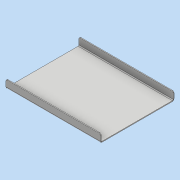
# Autodesk Inventor part: Schale
Saved by Autodesk Inventor 2018 (Build 220112000, 112)
## iProperties
Created: 2020-10-04
Part Number: Schale
Material: Generisch
Document SubType Name: Blech
Designer: marce
Density: 1 g/cm^3
Sheet Metal Rule: Standard_mm
Appearance: Vorgabe
Flat Pattern Width: 21.3048 cm
Flat Pattern Length: 23 cm
Flat Pattern Area: 490.01 cm^2
Sheet Metal Width: 213.048 mm
Sheet Metal Length: 230.000 mm
Sheet Metal Area: 49000.991 mm^2
Author: marce
Autodesk Inventor part; units mm, degrees
ref_plane "YZ Plane" through (0, 0, 0) normal (1, 0, 0) x (0, 1, 0)
ref_plane "XZ Plane" through (0, 0, 0) normal (0, 1, 0) x (-1, 0, 0)
ref_plane "XY Plane" through (0, 0, 0) normal (0, 0, 1) x (1, 0, 0)
sketch "Skizze1" plane through (0, 0, 0) normal (0, 0, 1) x (1, 0, 0)
  line L0 (0, 0) -> (230, 0)
  line L1 (230, 0) -> (230, 180)
  line L2 (230, 180) -> (0, 180)
  line L3 (0, 180) -> (0, 0)
  dimension "d0" = 230
  dimension "d1" = 180
  measures "d0" distance of L2.end L1.end
  measures "d1" distance of L1.end L0.end
extrude "Grobblech1" add sketch "Skizze1" along normal blind 2
sketch "Skizze2" plane through (230, 2, 0) normal (0, -1, 0) x (1, 0, 0)
  line L0 (-230, 0) -> (0, 0)
  line L1 (0, 0) -> (0, 20)
  line L2 (0, 20) -> (-230, 20)
  line L3 (-230, 20) -> (-230, 0)
  constraints: 6 end point, 1 horizontal, 1 perpendicular, 1 vertical
edge flange "Lasche1" height 20 angle 90 thickness 2 bend radius 2 thickness toward (0, -1, 0) relief straight relief width 2 relief depth 1 corner gap 2 corner form 0 edges at (115, 0, 2) (115, 180, 2) wall of the first edge with corners at (0, 2, 0) (230, 2, 0) (230, 2, 20) (0, 2, 20)
bend "Biegung1"
corner "Ecke1"
fillet "Eckenrundung1" radius 3 4 edges at (0, 1, 20) (0, 179, 20) (230, 179, 20) (230, 1, 20)
equation "\"d2\" = Stärke"
equation "\"d3\" = BreiteBiegungsfreistellung"
equation "\"d4\" = TiefeBiegungsfreistellung"
equation "\"d5\" = MinimalRest"
equation "\"d6\" = Übergangsradius"
equation "\"d9\" = Biegeradius"
equation "\"d10\" = GrößeEckenfreistellung"
equation "\"d11\" = Abstandsgröße"
equation "\"d12\" = JacobiRadiusGröße"
equation "\"Biegeradius\" = Stärke"
equation "\"BreiteBiegungsfreistellung\" = Stärke"
equation "\"TiefeBiegungsfreistellung\" = 0.5 * Stärke"
equation "\"GrößeEckenfreistellung\" = 4 * Stärke"
equation "\"MinimalRest\" = 2 * Stärke"
equation "\"Übergangsradius\" = Biegeradius"
equation "\"JacobiRadiusGröße\" = Biegeradius"
equation "\"Abstandsgröße\" = Stärke"
equation "\"Stärke\" = 2"
